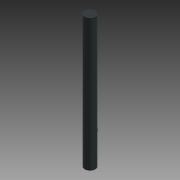
# Autodesk Inventor part: 1231_Spool Shaft_V1
Saved by Autodesk Inventor 2020 (Build 240168000, 168)
## iProperties
Created: 2019-09-13
Part Number: 1231_Spool Shaft_V1
Material: Iron, Ductile
Document SubType Name: Modeling
Designer: MPI
Density: 7.15 g/cm^3
Appearance: Iron Gray
Mass: 522.885 g
Surface Area: 575.556 cm^2
Volume: 522.885 cm^3
Author: MPI
Autodesk Inventor part; units mm, degrees
ref_plane "YZ Plane" through (0, 0, 0) normal (1, 0, 0) x (0, 1, 0)
ref_plane "XY Plane" through (0, 0, 0) normal (0, 0, 1) x (1, 0, 0)
sketch "Sketch1" plane through (0, 0, 0) normal (0, 0, 1) x (1, 0, 0)
  circle A0 centre (0, 0) radius 19.05
  dimension "d0" = 38.1
  constraints: 1 centre point, 1 coincident
  measures "d0" diameter of A0
extrude "Extrusion1" add sketch "Sketch1" along normal blind 480
ref_plane "Work Plane1" through (0, 15, 0) normal (0, 1, 0) x (-1, 0, 0)
sketch "Sketch2" plane through (0, 15, 0) normal (0, 1, 0) x (-1, 0, 0)
  line L0 (-122.6999, 230) -> (112.1399, 230) construction
  line L1 (-19.05, 0) -> (19.05, 0) projected
  line L2 (-122.6999, 128) -> (109.8048, 128) construction
  line L3 (-29.6313, 106) -> (33.0816, 106)
  line L4 (33.0816, 106) -> (33.0816, 118)
  line L5 (33.0816, 118) -> (-29.6313, 118)
  line L6 (-29.6313, 118) -> (-29.6313, 106)
  line L7 (-41.3065, 342) -> (43.7561, 342)
  line L8 (43.7561, 342) -> (43.7561, 354)
  line L9 (43.7561, 354) -> (-41.3065, 354)
  line L10 (-41.3065, 354) -> (-41.3065, 342)
  point P0 (0, 0)
  dimension "d5" = 230
  dimension "d6" = 102
  dimension "d8" = 12
  dimension "d9" = 12
  dimension "d11" = 112
  dimension "d14" = 112
  constraints: 20 end point, 4 horizontal, 4 parallel, 2 perpendicular
  measures "d5" distance between parallel lines of L0 L1
  measures "d6" distance between parallel lines of L0 L2
  measures "d8" distance of L5.end L3.start
  measures "d9" distance of L9.end L7.start
  measures "d11" distance between parallel lines of L7 L0
  measures "d14" distance between parallel lines of L5 L0
extrude "Extrusion2" cut sketch "Sketch2" along normal through all
body "Solid1"
